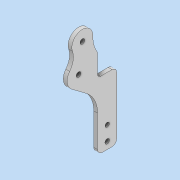
# Autodesk Inventor part: Kettenblech_zusatz
Saved by Autodesk Inventor 2022 (Build 260153000, 153)
## iProperties
Created: 2021-04-15
Part Number: Kettenblech_zusatz
Material: Generic
Document SubType Name: Modeling
Designer: Fabijan_Sven
Density: 1 g/cm^3
Appearance: Default
Author: Fabijan_Sven
Autodesk Inventor part; units mm, degrees
ref_plane "YZ Plane" through (0, 0, 0) normal (1, 0, 0) x (0, 1, 0)
ref_plane "XZ Plane" through (0, 0, 0) normal (0, 1, 0) x (-1, 0, 0)
ref_plane "XY Plane" through (0, 0, 0) normal (0, 0, 1) x (1, 0, 0)
sketch "Sketch1" plane through (0, 0, 0) normal (1, 0, 0) x (0, 1, 0)
  line L0 (-60.7701, 7.4226) -> (-60.7701, -12.5774)
  line L1 (-60.7701, -12.5774) -> (9.2299, -12.5774)
  line L2 (9.2299, -12.5774) -> (9.2299, 7.4226)
  circle A0 centre (50.2299, 23.4226) radius 2.5
  line L3 (12.2299, 7.4226) -> (-387.7701, 7.4226) projected
  line L4 (32.2299, -27.5774) -> (32.23, -2.5774) projected
  line L5 (12.2299, 7.4226) -> (12.2299, -492.5774) projected
  line L6 (32.23, -2.5774) -> (32.2299, 7.4226)
  line L7 (9.2299, 7.4226) -> (32.2299, 7.4226)
  arc A1 (50.2299, 12.4226) -> (46.5993, 33.8061) centre (50.2299, 23.4226) ccw projected
  arc A2 (50.2299, 12.4226) -> (32.23, -2.5774) centre (50.2299, -5.8774) ccw projected
  arc A3 (29.7933, 36.739) -> (46.5993, 33.8061) centre (40.8232, 50.3254) ccw projected
  arc A4 (29.7933, 36.739) -> (12.6299, 34.6226) centre (22.2299, 27.4226) ccw projected
  line L8 (12.6299, 34.6226) -> (-6.7701, 8.7559) projected
  arc A5 (49.5524, 12.4435) -> (46.5993, 33.8061) centre (50.2299, 23.4226) ccw
  arc A6 (29.7933, 36.739) -> (12.6299, 34.6226) centre (22.2299, 27.4226) ccw
  arc A7 (29.7933, 36.739) -> (46.5993, 33.8061) centre (40.8232, 50.3254) ccw
  line L9 (12.6299, 34.6226) -> (-7.7701, 7.4226)
  circle A8 centre (22.2299, 27.4226) radius 2.5
  arc A9 (50.2299, 12.4226) -> (32.2299, 7.4226) centre (48.9563, -17.8924) ccw
  line L10 (-7.7701, 7.4226) -> (-60.7701, 7.4226)
  point P0 (0, 0)
  point P1 (12.2299, 7.4226)
  point P2 (32.23, -2.5774)
  point P3 (50.2299, 12.4226)
  point P4 (50.2299, 12.4226)
  dimension "d6" = 70
  dimension "d7" = 3
  dimension "d8" = 0
  dimension "d19" = 5
  dimension "d20" = 5
  dimension "d21" = 30.3417
  constraints: 14 end point, 9 point on circle, 6 centre point, 5 coincident, 4 point on line, 3 horizontal, 2 parallel, 1 concentric, 1 perpendicular, 1 tangent, 5 other
  measures "d6" distance between parallel lines of L0 L2
  measures "d7" distance between parallel lines of L2 L5
  measures "d8" distance of L7.start L2.end
  measures "d19" diameter of A0
  measures "d20" diameter of A8
  measures "d21" radius of A9
extrude "Extrusion1" add sketch "Sketch1" along normal blind 4 contours L3 L2 L1 L0 | L9 L8 A4 A3 A1 A9 L7 L3
fillet "Fillet1" radius 5 4 edges at (2, 32.2299, 7.4226) (2, 9.2299, -12.5774) (2, -60.7701, -12.5774) (2, -60.7701, 7.4226)
fillet "Fillet2" radius 3 1 edges at (2, 9.2299, 7.4226)
sketch "Sketch2" plane through (4, 0, 0) normal (1, 0, 0) x (0, 0, -1)
  circle A0 centre (2.5774, -38.2701) radius 2.255
  circle A1 centre (2.5774, -53.2701) radius 2.3918
  line L0 (12.5774, -55.7701) -> (12.5774, 4.2299) projected
  line L1 (-2.4226, -60.7701) -> (7.5774, -60.7701) projected
  line L2 (7.5774, 9.2299) -> (-4.4226, 9.2299) projected
  point P0 (0, 0)
  dimension "d13" = 10
  dimension "d14" = 10
  dimension "d15" = 7.5
  dimension "d16" = 47.5
  constraints: 2 centre point
  measures "d13" distance from line of L0 A0.centre
  measures "d14" distance from line of L0 A1.centre
  measures "d15" distance from line of A1.centre L1
  measures "d16" distance from line of A0.centre L2
extrude "Extrusion2" cut sketch "Sketch2" against normal blind 10
fillet "Fillet3" radius 30 1 edges at (2, -7.7701, 7.4226)
body "Solid1"
